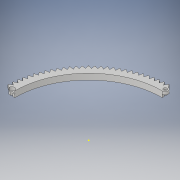
# Autodesk Inventor part: Bevel_Inner_gear1_4
Saved by Autodesk Inventor 2019 (Build 230136000, 136)
## iProperties
Created: 2019-05-19
Part Number: Bevel_Inner_gear1_4
Material: Generic
Document SubType Name: Modeling
Designer: Jorian Brusind
Density: 1 g/cm^3
Appearance: Default
Author: Jorian Brusind
Autodesk Inventor part; units mm, degrees
note: some values were not read from the file. Chosen so that the rebuilt part matches the saved one: pattern direction of "Circular Pattern2".
ref_plane "YZ Plane" through (0, 0, 0) normal (1, 0, 0) x (0, 1, 0)
ref_plane "XZ Plane" through (0, 0, 0) normal (0, 1, 0) x (-1, 0, 0)
ref_plane "XY Plane" through (0, 0, 0) normal (0, 0, 1) x (1, 0, 0)
sketch "Sketch1" plane through (0, 0, 0) normal (0, 1, 0) x (-1, 0, 0)
  line L0 (0, 0) -> (0, -125) construction
  line L1 (0, 0) -> (125, 0) construction
  arc A0 (0, -135) -> (135, 0) centre (0, 0) ccw
  line L2 (125, 0) -> (135, 0)
  line L3 (0, -135) -> (0, -125)
  arc A1 (0, -125) -> (125, 0) centre (0, 0) ccw
  dimension "d1" = 90
  dimension "d2" = 135
  dimension "d3" = 125
  constraints: 8 end point, 4 point on circle, 3 coincident, 2 centre point, 2 horizontal, 2 perpendicular
  measures "d1" angle of L0 L1
  measures "d2" radius of A0
  measures "d3" radius of A1
extrude "Extrusion1" add sketch "Sketch1" along normal blind 10
sketch "Sketch2" plane through (0, 10, 0) normal (0, 1, 0) x (1, 0, 0)
  line L0 (-135, 0) -> (-125, 0) projected
  circle A0 centre (-130, 0) radius 2.5
  arc A1 (0, 135) -> (-135, 0) centre (0, 0) ccw projected
  circle A2 centre (-130, 0) radius 5
  line L1 (-130, 0) -> (0, 0)
  dimension "d6" = 5
  constraints: 2 end point, 1 centre point, 1 coincident, 1 horizontal, 1 horizontal alignment, 1 midpoint, 2 other
  measures "d6" diameter of A0
extrude "Extrusion2" cut sketch "Sketch2" against normal blind 5
sketch "Sketch3" plane through (0, 0, 0) normal (0, -1, 0) x (1, 0, 0)
  point P0 (0, 0)
sketch "Sketch4" plane through (0, 10, 0) normal (0, 1, 0) x (1, 0, 0)
  line L0 (0, 125) -> (0, 135) projected
  circle A0 centre (0, 130) radius 5
  point P0 (0, 0)
  constraints: 1 midpoint, 1 vertical alignment, 2 other
extrude "Extrusion3" add sketch "Sketch4" against normal blind 5
sketch "Sketch5" plane through (0, 10, 0) normal (0, 1, 0) x (1, 0, 0)
  line L0 (0, 125) -> (0, 135) projected
  circle A0 centre (0, 130) radius 1.75
  line L1 (-135, 0) -> (-125, 0) projected
  circle A1 centre (-130, 0) radius 1.75
  point P0 (0, 0)
  dimension "d11" = 3.5
  dimension "d12" = 3.5
  constraints: 2 centre point, 2 midpoint
  measures "d11" diameter of A0
  measures "d12" diameter of A1
extrude "Extrusion4" cut sketch "Sketch5" against normal blind 10
sketch "Sketch6" plane through (0, 10, 0) normal (0, 1, 0) x (1, 0, 0)
  line L0 (0, 0) -> (-95.459415, 95.459415)
  arc A0 (0, 135) -> (-135, 0) centre (0, 0) ccw
  line L1 (0, 0) -> (135, 0) construction
  line L2 (-95.459415, 95.459415) -> (-92.984542, 97.934289)
  line L3 (-95.459415, 95.459415) -> (-97.934289, 92.984542)
  line L4 (-95.459415, 95.459415) -> (-91.959415, 95.459415) construction
  line L5 (-95.459415, 95.459415) -> (-98.994949, 98.994949)
  line L6 (-98.994949, 98.994949) -> (-99.348503, 98.641396)
  line L7 (-98.994949, 98.994949) -> (-98.641396, 99.348503)
  line L8 (-99.348503, 98.641396) -> (-97.934289, 92.984542)
  line L9 (-98.641396, 99.348503) -> (-92.984542, 97.934289)
  line L10 (-95.459415, 95.459415) -> (-102.323655, 88.061738)
  line L11 (-97.934289, 92.984542) -> (-102.323655, 88.061738)
  line L12 (-95.459415, 95.459415) -> (-92.952881, 97.901797)
  line L13 (-92.984542, 97.934289) -> (-92.952881, 97.901797)
  dimension "d15" = 135
  dimension "d16" = 3.5
  dimension "d17" = 3.5
  dimension "d18" = 135
  dimension "d19" = 5
  dimension "d20" = 0.5
  dimension "d21" = 0.5
  dimension "d22" = 135
  dimension "d23" = 90
  dimension "d24" = 10.09175
  constraints: 28 end point, 3 perpendicular, 3 point on circle, 2 equal length, 2 horizontal, 2 tangent
  measures "d15" angle of L1 L0
  measures "d16" distance of L0.end L2.end
  measures "d17" distance of L0.end L3.end
  measures "d18" angle of L3 L4
  measures "d19" distance of L0.end L5.end
  measures "d20" distance of L5.end L6.end
  measures "d21" distance of L5.end L7.end
  measures "d22" angle of L4 L5
  measures "d23" angle of L5 L7
  measures "d24" distance of L0.end L10.end
extrude "Extrusion5" add sketch "Sketch6" against normal blind 5 contours A0 L2 L13 | L10 L11 A0 | L5 L7 L9 L2 | A0 L11 L3 | L3 L8 L6 L5
sketch "Sketch8" plane through (0, 10, 0) normal (0, 1, 0) x (1, 0, 0)
  circle A0 centre (0, 130) radius 1.75 projected
  circle A1 centre (0, 130) radius 3
  point P0 (0, 0)
  dimension "d32" = 6
  constraints: 1 centre point, 1 coincident
  measures "d32" diameter of A1
extrude "Extrusion7" cut sketch "Sketch8" against normal blind 3
pattern_circular "Circular Pattern2" count 30 over 90 about axis through (0, 0, 0) along (0, 1, 0) of "Extrusion5" both ways yes
sketch "Sketch12" plane through (0, 10, 0) normal (0, 1, 0) x (1, 0, 0)
  line L0 (-139.9622, 0) -> (-121.238538, 0)
  line L1 (-121.238538, 0) -> (-121.238538, -17.107219)
  line L2 (-121.238538, -17.107219) -> (-139.9622, -17.107219)
  line L3 (-139.9622, -17.107219) -> (-139.9622, 0)
  point P0 (0, 0)
  constraints: 8 end point, 2 parallel, 1 horizontal, 1 perpendicular
extrude "Extrusion12" cut sketch "Sketch12" against normal blind 10
body "Solid1"
